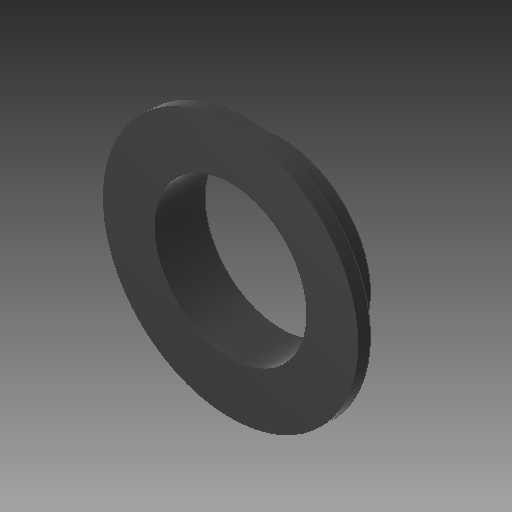
# Autodesk Inventor part: オイレスF 12-14 3t
Saved by Autodesk Inventor 2017.3 (Build 213256000, 256)
## iProperties
Part Number: オイレスF 12-14 3t
Material: アセタール樹脂、黒
Document SubType Name: Modeling
Designer: 原知也
Density: 1.425 g/cm^3
Appearance: 滑らか - 黒
Mass: 0.461107 g
Surface Area: 7.47699 cm^2
Volume: 0.323584 cm^3
Author: 原知也
Autodesk Inventor part; units mm, degrees
ref_plane "YZ Plane" through (0, 0, 0) normal (1, 0, 0) x (0, 1, 0)
ref_plane "XZ Plane" through (0, 0, 0) normal (0, 1, 0) x (-1, 0, 0)
ref_plane "XY Plane" through (0, 0, 0) normal (0, 0, 1) x (1, 0, 0)
sketch "スケッチ1" plane through (0, 0, 0) normal (0, 0, 1) x (1, 0, 0)
  circle A0 centre (0, 0) radius 6
  circle A1 centre (0, 0) radius 7
  dimension "d0" = 12
  dimension "d1" = 14
  constraints: 2 centre point, 2 coincident
  measures "d0" diameter of A0
  measures "d1" diameter of A1
extrude "押し出し1" add sketch "スケッチ1" along normal blind 3
sketch "スケッチ2" plane through (0, 0, 3) normal (0, 0, 1) x (1, 0, 0)
  circle A0 centre (0, 0) radius 6 projected
  circle A1 centre (0, 0) radius 10
  dimension "d4" = 20
  constraints: 1 centre point, 1 coincident
  measures "d4" diameter of A1
extrude "押し出し2" add sketch "スケッチ2" along normal blind 1
